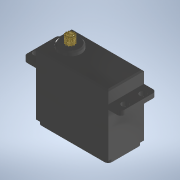
# Autodesk Inventor part: MG996R Servo
Saved by Autodesk Inventor 2021 (Build 250183000, 183)
## iProperties
Created: 2017-08-15
Part Number: MG996R Servo
Material: ABS Plastic
Document SubType Name: Modeling
Designer: Izuwa
Density: 1.06 g/cm^3
Appearance: Smooth - White
Mass: 31.0362 g
Surface Area: 66.5216 cm^2
Volume: 29.2795 cm^3
Author: Izuwa
Autodesk Inventor part; units mm, degrees
ref_plane "YZ Plane" through (0, 0, 0) normal (1, 0, 0) x (0, 1, 0)
ref_plane "XZ Plane" through (0, 0, 0) normal (0, 1, 0) x (-1, 0, 0)
ref_plane "XY Plane" through (0, 0, 0) normal (0, 0, 1) x (1, 0, 0)
sketch "Sketch1" plane through (0, 0, 0) normal (0, 0, 1) x (1, 0, 0)
  line L0 (0, 0) -> (40, 0)
  line L1 (40, 0) -> (40, 19.82)
  line L2 (40, 19.82) -> (0, 19.82)
  line L3 (0, 19.82) -> (0, 0)
  dimension "d1" = 19.82
  dimension "d53" = 40
  constraints: 8 end point, 2 parallel, 1 horizontal, 1 perpendicular
  measures "d1" distance of L1.end L0.end
  measures "d53" distance of L1.end L2.end
extrude "Extrusion1" add sketch "Sketch1" along normal blind 26.67
sketch "Sketch2" plane through (0, 0, 26.67) normal (0, 0, 1) x (1, 0, 0)
  line L0 (40, 0) -> (40, 19.82) projected
  line L1 (0, 0) -> (40, 0)
  line L2 (40, 0) -> (40, 19.82)
  line L3 (40, 19.82) -> (0, 19.82)
  line L4 (0, 19.82) -> (0, 0)
  line L5 (-7, 19.82) -> (47, 19.82)
  line L6 (47, 19.82) -> (47, 0)
  line L7 (47, 0) -> (-7, 0)
  line L8 (-7, 0) -> (-7, 19.82)
  line L9 (40, 19.82) -> (0, 19.82) projected
  line L10 (0, 0) -> (40, 0) projected
  line L11 (0, 19.82) -> (0, 0) projected
  line L12 (0, 9.91) -> (40, 9.91)
  line L13 (20, 22.239) -> (20, -2.7088)
  point P0 (20, 19.82)
  dimension "d56" = 20
  dimension "d57" = 54
  constraints: 20 end point, 4 parallel, 3 midpoint, 3 point on line, 2 horizontal, 2 perpendicular, 1 vertical
  measures "d56" distance between parallel lines of L0 L13
  measures "d57" distance between parallel lines of L6 L8
extrude "Extrusion2" add sketch "Sketch2" along normal blind 2.5
sketch "Sketch3" plane through (0, 0, 29.17) normal (0, 0, 1) x (1, 0, 0)
  line L0 (0, 0) -> (40, 0) projected
  line L1 (40, 19.82) -> (0, 19.82) projected
  line L2 (0, 0) -> (40, 0)
  line L3 (40, 0) -> (40, 19.82)
  line L4 (40, 19.82) -> (0, 19.82)
  line L5 (0, 19.82) -> (0, 0)
  constraints: 8 end point, 2 parallel, 1 horizontal, 1 perpendicular
extrude "Extrusion3" add sketch "Sketch3" along normal blind 6.85
sketch "Sketch8" plane through (0, 0, 29.17) normal (0, 0, 1) x (1, 0, 0)
  line L0 (0, 19.82) -> (0, 0) projected
  line L1 (40, 0) -> (40, 19.82) projected
  circle A0 centre (-4.5, 14.91) radius 1.9
  circle A1 centre (-4.5, 4.91) radius 1.9
  circle A2 centre (44.5, 14.91) radius 1.9
  circle A3 centre (44.5, 4.91) radius 1.9
  line L2 (9.66, 9.91) -> (9.66, 35.2496)
  line L3 (47, 0) -> (47, 19.82) projected
  line L4 (-7, 0) -> (-7, 19.82) projected
  line L5 (-7, 9.91) -> (-13.5914, 9.91)
  dimension "d47" = 3.8
  dimension "d48" = 3.8
  dimension "d49" = 3.8
  dimension "d52" = 9.66
  dimension "d54" = 4.5
  dimension "d55" = 7
  dimension "d58" = 4.5
  dimension "d59" = 2.5
  dimension "d60" = 2.5
  constraints: 4 centre point, 4 end point, 1 horizontal, 1 midpoint, 1 vertical
  measures "d47" diameter of A1
  measures "d48" diameter of A2
  measures "d49" diameter of A3
  measures "d52" distance between parallel lines of L0 L2
  measures "d54" distance from line of L1 A2.centre
  measures "d55" distance between parallel lines of L1 L3
  measures "d58" distance from line of A0.centre L0
  measures "d59" distance from line of L3 A3.centre
  measures "d60" distance from line of L3 A2.centre
extrude "Extrusion8" cut sketch "Sketch8" against normal blind 777
sketch "Sketch4" plane through (0, 0, 36.02) normal (0, 0, 1) x (1, 0, 0)
  line L0 (0, 0) -> (40, 0) projected
  line L1 (40, 0) -> (40, 19.82) projected
  line L2 (0, 0) -> (40, 0)
  line L3 (40, 0) -> (40, 19.82)
  line L4 (40, 19.82) -> (0, 19.82)
  line L5 (0, 19.82) -> (0, 0)
  line L6 (0, 0) -> (0, 19.82) projected
  circle A0 centre (8.97, 9.91) radius 6
  circle A1 centre (-4.5, 14.91) radius 1.9 projected
  dimension "d74" = 13.47
  constraints: 8 end point, 2 parallel, 1 centre point, 1 horizontal, 1 perpendicular
  measures "d74" horizontal distance of A1.centre A0.centre
extrude "Extrusion4" add sketch "Sketch4" along normal blind 2.33 contours A0
sketch "Sketch5" plane through (8.97, 9.91, 38.35) normal (0, 0, 1) x (1, 0, 0)
  circle A0 centre (0, 0) radius 2.5
  point P0 (-8.97, -9.91)
  dimension "d13" = 5
  constraints: 1 centre point
  measures "d13" diameter of A0
extrude "Extrusion5" add sketch "Sketch5" along normal blind 4.05
sketch "Sketch6" plane through (8.97, 9.91, 42.4) normal (0, 0, 1) x (1, 0, 0)
  line L0 (2.0681, 0.3647) -> (2.4905, 0.2179)
  line L1 (1.9734, 0.7182) -> (2.2658, 1.0565)
  arc A0 (2.0681, 0.3647) -> (1.9734, 0.7182) centre (0, 0) ccw
  arc A1 (0.2179, 2.4905) -> (0, 2.5) centre (0, 0) ccw
  arc A2 (2.4905, 0.2179) -> (2.2658, 1.0565) centre (0, 0) ccw
  point P0 (-8.97, -9.91)
  constraints: 6 point on circle, 4 end point, 3 centre point, 1 coincident
extrude "Extrusion6" cut sketch "Sketch6" against normal blind 4.05
pattern_circular "Circular Pattern1" count 12 over 360 about axis through (8.97, 9.91, 38.35) along (0, 0, 1) of "Extrusion6"
sketch "Sketch7" plane through (0, 0, 0) normal (0, 0, -1) x (-1, 0, 0)
  line L0 (-40, 0) -> (-40, 19.82) projected
  line L1 (0, 0) -> (-40, 0)
  line L2 (-40, 0) -> (-40, 19.82)
  line L3 (-40, 19.82) -> (0, 19.82)
  line L4 (0, 19.82) -> (0, 0)
  line L5 (-39.5, 0.5) -> (-0.5, 0.5)
  line L6 (-0.5, 0.5) -> (-0.5, 19.32)
  line L7 (-0.5, 19.32) -> (-39.5, 19.32)
  line L8 (-39.5, 19.32) -> (-39.5, 0.5)
  dimension "d29" = 0.5
  constraints: 16 end point, 4 parallel, 2 perpendicular, 1 horizontal, 3 other
  measures "d29" distance between parallel lines of L1 L5
extrude "Extrusion7" cut sketch "Sketch7" against normal blind 2
fillet "Fillet1" radius 2 4 edges at (39.5, 0.5, 1) (39.5, 19.32, 1) (0.5, 0.5, 1) (0.5, 19.32, 1)
sketch "Sketch9" plane through (8.97, 9.91, 42.4) normal (0, 0, 1) x (1, 0, 0)
  circle A0 centre (0, 0) radius 1
  point P0 (-8.97, -9.91)
  dimension "d61" = 2
  constraints: 1 centre point
  measures "d61" diameter of A0
extrude "Extrusion9" cut sketch "Sketch9" against normal blind 5
chamfer "Chamfer1" distance 0.7 angle 45 1 edges at (7.97, 9.91, 42.4)
fillet "Fillet2" radius 2 4 edges at (47, 0, 27.92) (47, 19.82, 27.92) (-7, 19.82, 27.92) (-7, 0, 27.92)
chamfer "Chamfer2" distance 0.7 angle 45 1 edges at (2.97, 9.91, 38.35)
chamfer "Chamfer3" distance 0.7 angle 45 4 edges at (40, 9.91, 36.02) (20, 0, 36.02) (20, 19.82, 36.02) (0, 9.91, 36.02)
sketch "Sketch10" plane through (0, 0, 36.02) normal (0, 0, 1) x (1, 0, 0)
  arc A0 (-7, 2) -> (-5, 0) centre (-5, 2) ccw projected
  line L0 (-5, 0) -> (0, 0) projected
  line L1 (0, 0) -> (0, 19.82) projected
  line L2 (0, 19.82) -> (-5, 19.82) projected
  arc A1 (-5, 19.82) -> (-7, 17.82) centre (-5, 17.82) ccw projected
  line L3 (-7, 17.82) -> (-7, 2) projected
  circle A2 centre (-4.5, 14.91) radius 1.9 projected
  circle A3 centre (-4.5, 4.91) radius 1.9 projected
  circle A4 centre (44.5, 4.91) radius 1.9 projected
  circle A5 centre (44.5, 14.91) radius 1.9 projected
  arc A6 (47, 17.82) -> (45, 19.82) centre (45, 17.82) ccw projected
  line L4 (45, 19.82) -> (40, 19.82) projected
  line L5 (40, 19.82) -> (40, 0) projected
  line L6 (40, 0) -> (45, 0) projected
  arc A7 (45, 0) -> (47, 2) centre (45, 2) ccw projected
  line L7 (47, 2) -> (47, 17.82) projected
  line L8 (40, 19.82) -> (0, 19.82) projected
  line L9 (0, 0) -> (40, 0) projected
  circle A8 centre (8.97, 9.91) radius 6 projected
  line L10 (0.7, 0.7) -> (0.7, 19.12) projected
  line L11 (39.3, 0.7) -> (0.7, 0.7) projected
  line L12 (39.3, 19.12) -> (39.3, 0.7) projected
  line L13 (0.7, 19.12) -> (39.3, 19.12) projected
ref_plane "Work Plane1" through (47, 2, 26.67) normal (1, 0, 0) x (0, 0, -1)
sketch "Sketch13" plane through (0, 0, 2) normal (0, -1, 0) x (1, 0, 0)
  line L0 (19.97, 43.17) -> (-2.03, 43.17) projected
  line L1 (19.97, 43.17) -> (19.97, 40.4)
  line L2 (-2.03, 43.17) -> (-2.03, 40.4)
  line L3 (39.3, 34.02) -> (0.7, 34.02) projected
  line L4 (-5, 27.17) -> (0, 27.17) projected
  line L5 (40, 27.17) -> (45, 27.17) projected
  line L6 (0, 33.32) -> (40, 33.32) projected
  line L7 (0, 27.17) -> (0, 33.32) projected
  line L8 (-5, 27.17) -> (0, 27.17) projected
  line L9 (-5, 24.67) -> (-5, 27.17) projected
  line L10 (0, 24.67) -> (-5, 24.67) projected
  line L11 (0, 0) -> (0, 24.67) projected
  line L12 (0, 0) -> (40, 0) projected
  line L13 (40, 0) -> (40, 24.67) projected
  line L14 (45, 24.67) -> (40, 24.67) projected
  line L15 (45, 27.17) -> (45, 24.67) projected
  line L16 (40, 27.17) -> (45, 27.17) projected
  line L17 (40, 27.17) -> (40, 33.32) projected
  line L18 (37.5, -2) -> (2.5, -2) projected
  point P0 (0, -2)
  constraints: 4 end point, 2 vertical, 2 other
sketch "Sketch14" plane through (0, 0, 36.02) normal (0, 0, 1) x (1, 0, 0)
  arc A0 (-7, 2) -> (-5, 0) centre (-5, 2) ccw projected
  line L0 (-5, 0) -> (0, 0) projected
  line L1 (0, 0) -> (0, 19.82) projected
  line L2 (0, 19.82) -> (-5, 19.82) projected
  arc A1 (-5, 19.82) -> (-7, 17.82) centre (-5, 17.82) ccw projected
  line L3 (-7, 17.82) -> (-7, 2) projected
  circle A2 centre (-4.5, 14.91) radius 1.9 projected
  circle A3 centre (-4.5, 4.91) radius 1.9 projected
  circle A4 centre (8.97, 9.91) radius 6 projected
  line L4 (0.7, 0.7) -> (0.7, 19.12) projected
  line L5 (39.3, 0.7) -> (0.7, 0.7) projected
  line L6 (39.3, 19.12) -> (39.3, 0.7) projected
  line L7 (0.7, 19.12) -> (39.3, 19.12) projected
  circle A5 centre (44.5, 4.91) radius 1.9 projected
  circle A6 centre (44.5, 14.91) radius 1.9 projected
  arc A7 (47, 17.82) -> (45, 19.82) centre (45, 17.82) ccw projected
  line L8 (45, 19.82) -> (40, 19.82) projected
  line L9 (40, 19.82) -> (40, 0) projected
  line L10 (40, 0) -> (45, 0) projected
  arc A8 (45, 0) -> (47, 2) centre (45, 2) ccw projected
  line L11 (47, 2) -> (47, 17.82) projected
sketch "Sketch16" plane through (0, 0, 0) normal (0, 0, -1) x (-1, 0, 0)
  arc A0 (-0.5, 17.32) -> (-2.5, 19.32) centre (-2.5, 17.32) ccw projected
  line L0 (-2.5, 19.32) -> (-37.5, 19.32) projected
  arc A1 (-37.5, 19.32) -> (-39.5, 17.32) centre (-37.5, 17.32) ccw projected
  line L1 (-39.5, 17.32) -> (-39.5, 2.5) projected
  arc A2 (-39.5, 2.5) -> (-37.5, 0.5) centre (-37.5, 2.5) ccw projected
  line L2 (-37.5, 0.5) -> (-2.5, 0.5) projected
  arc A3 (-2.5, 0.5) -> (-0.5, 2.5) centre (-2.5, 2.5) ccw projected
  line L3 (-0.5, 2.5) -> (-0.5, 17.32) projected
  circle A4 centre (-8.97, 9.91) radius 6 projected
  point P0 (0, 0)
sketch "Sketch18" plane through (0, 0, 36.02) normal (0, 0, 1) x (1, 0, 0)
  arc A0 (11.4605, 9.6921) -> (11.4605, 10.1279) centre (8.97, 9.91) ccw projected
  line L0 (11.0381, 9.5453) -> (11.4605, 9.6921) projected
  arc A1 (10.9434, 9.1918) -> (11.0381, 9.5453) centre (8.97, 9.91) ccw projected
  line L1 (11.2358, 8.8535) -> (10.9434, 9.1918) projected
  arc A2 (11.0179, 8.4761) -> (11.2358, 8.8535) centre (8.97, 9.91) ccw projected
  line L2 (10.5787, 8.5601) -> (11.0179, 8.4761) projected
  arc A3 (10.3199, 8.3013) -> (10.5787, 8.5601) centre (8.97, 9.91) ccw projected
  line L3 (10.4039, 7.8621) -> (10.3199, 8.3013) projected
  arc A4 (10.0265, 7.6442) -> (10.4039, 7.8621) centre (8.97, 9.91) ccw projected
  line L4 (9.6882, 7.9366) -> (10.0265, 7.6442) projected
  arc A5 (9.3347, 7.8419) -> (9.6882, 7.9366) centre (8.97, 9.91) ccw projected
  line L5 (9.1879, 7.4195) -> (9.3347, 7.8419) projected
  arc A6 (8.7521, 7.4195) -> (9.1879, 7.4195) centre (8.97, 9.91) ccw projected
  line L6 (8.6053, 7.8419) -> (8.7521, 7.4195) projected
  arc A7 (8.2518, 7.9366) -> (8.6053, 7.8419) centre (8.97, 9.91) ccw projected
  line L7 (7.9135, 7.6442) -> (8.2518, 7.9366) projected
  arc A8 (7.5361, 7.8621) -> (7.9135, 7.6442) centre (8.97, 9.91) ccw projected
  line L8 (7.6201, 8.3013) -> (7.5361, 7.8621) projected
  arc A9 (7.3613, 8.5601) -> (7.6201, 8.3013) centre (8.97, 9.91) ccw projected
  line L9 (6.9221, 8.4761) -> (7.3613, 8.5601) projected
  arc A10 (6.7042, 8.8535) -> (6.9221, 8.4761) centre (8.97, 9.91) ccw projected
  line L10 (6.9966, 9.1918) -> (6.7042, 8.8535) projected
  arc A11 (6.9019, 9.5453) -> (6.9966, 9.1918) centre (8.97, 9.91) ccw projected
  line L11 (6.4795, 9.6921) -> (6.9019, 9.5453) projected
  arc A12 (6.4795, 10.1279) -> (6.4795, 9.6921) centre (8.97, 9.91) ccw projected
  line L12 (6.9019, 10.2747) -> (6.4795, 10.1279) projected
  arc A13 (6.9966, 10.6282) -> (6.9019, 10.2747) centre (8.97, 9.91) ccw projected
  line L13 (6.7042, 10.9665) -> (6.9966, 10.6282) projected
  arc A14 (6.9221, 11.3439) -> (6.7042, 10.9665) centre (8.97, 9.91) ccw projected
  line L14 (7.3613, 11.2599) -> (6.9221, 11.3439) projected
  arc A15 (7.6201, 11.5187) -> (7.3613, 11.2599) centre (8.97, 9.91) ccw projected
  line L15 (7.5361, 11.9579) -> (7.6201, 11.5187) projected
  arc A16 (7.9135, 12.1758) -> (7.5361, 11.9579) centre (8.97, 9.91) ccw projected
  line L16 (8.2518, 11.8834) -> (7.9135, 12.1758) projected
  arc A17 (8.6053, 11.9781) -> (8.2518, 11.8834) centre (8.97, 9.91) ccw projected
  line L17 (8.7521, 12.4005) -> (8.6053, 11.9781) projected
  arc A18 (9.1879, 12.4005) -> (8.7521, 12.4005) centre (8.97, 9.91) ccw projected
  line L18 (9.3347, 11.9781) -> (9.1879, 12.4005) projected
  arc A19 (9.6882, 11.8834) -> (9.3347, 11.9781) centre (8.97, 9.91) ccw projected
  line L19 (10.0265, 12.1758) -> (9.6882, 11.8834) projected
  arc A20 (10.4039, 11.9579) -> (10.0265, 12.1758) centre (8.97, 9.91) ccw projected
  line L20 (10.3199, 11.5187) -> (10.4039, 11.9579) projected
  arc A21 (10.5787, 11.2599) -> (10.3199, 11.5187) centre (8.97, 9.91) ccw projected
  line L21 (11.0179, 11.3439) -> (10.5787, 11.2599) projected
  arc A22 (11.2358, 10.9665) -> (11.0179, 11.3439) centre (8.97, 9.91) ccw projected
  line L22 (10.9434, 10.6282) -> (11.2358, 10.9665) projected
  arc A23 (11.0381, 10.2747) -> (10.9434, 10.6282) centre (8.97, 9.91) ccw projected
  line L23 (11.4605, 10.1279) -> (11.0381, 10.2747) projected
  circle A24 centre (8.97, 9.91) radius 5.3 projected
  line L24 (8.97, 9.91) -> (8.97, -8.7345)
  circle A25 centre (8.97, 9.91) radius 1 projected
  line L25 (8.97, 9.91) -> (3.5332, -10.3804)
  line L26 (8.97, 9.91) -> (14.317, -10.0453)
  point P0 (0, 0)
  dimension "d83" = 15
  dimension "d84" = 15
  constraints: 6 end point, 1 vertical
  measures "d83" angle of L24 L26
  measures "d84" angle of L25 L24
sketch "Sketch19" plane through (0, 0, 0) normal (0, 0, -1) x (-1, 0, 0)
  line L0 (-8.97, 9.91) -> (-3.5332, -10.3804) projected
  line L1 (-8.97, 9.91) -> (-14.317, -10.0453) projected
  point P0 (0, 0)
ref_plane "Work Plane2" through (8.97, 9.91, 36.02) normal (0.9659258, 0.258819, 0) x (0.258819, -0.9659258, 0)
ref_plane "Work Plane3" through (8.97, 9.91, 36.02) normal (0.9659258, -0.258819, 0) x (-0.258819, -0.9659258, 0)
body "Solid1"
